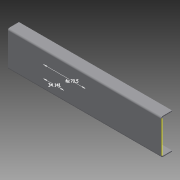
# Autodesk Inventor part: crane_lower
Saved by Autodesk Inventor 2014 SP2 (Build 180246200, 246)
## iProperties
Created: 2016-04-26
Part Number: crane_lower
Material: Generic
Document SubType Name: Sheet Metal
Designer: cruiser
Density: 1 g/cm^3
Flat Pattern Width: 9.17817 cm
Flat Pattern Length: 25.8 cm
Flat Pattern Area: 236.797 cm^2
Sheet Metal Rule: Default_mm
Sheet Metal Width: 91.782 mm
Sheet Metal Length: 258.000 mm
Sheet Metal Area: 23679.674 mm^2
Appearance: Default
Author: cruiser
Autodesk Inventor part; units mm, degrees
ref_plane "YZ Plane" through (0, 0, 0) normal (1, 0, 0) x (0, 1, 0)
ref_plane "XZ Plane" through (0, 0, 0) normal (0, 1, 0) x (-1, 0, 0)
ref_plane "XY Plane" through (0, 0, 0) normal (0, 0, 1) x (1, 0, 0)
sketch "Sketch1" plane through (0, 0, 0) normal (0, 1, 0) x (-1, 0, 0)
  line L0 (70.5, -70.5) -> (-70.5, -70.5)
  line L1 (-70.5, -70.5) -> (-70.5, 70.5)
  line L2 (-70.5, 70.5) -> (70.5, 70.5)
  line L3 (70.5, 70.5) -> (70.5, -70.5)
  line L4 (70.5, -70.5) -> (-70.5, 70.5) construction
  line L5 (-70.5, -70.5) -> (70.5, 70.5) construction
  line L6 (129, -30) -> (-129, -30)
  line L7 (-129, -30) -> (-129, 30)
  line L8 (-129, 30) -> (129, 30)
  line L9 (129, 30) -> (129, -30)
  line L10 (129, -30) -> (-129, 30) construction
  line L11 (-129, -30) -> (129, 30) construction
  point P0 (0, 0)
  dimension "d0" = 258
  dimension "d1" = 60
  dimension "d2" = 141
  dimension "d3" = 141
  measures "d0" distance of L6.start L6.end
  measures "d1" distance of L6.end L7.end
  measures "d2" distance of L0.start L0.end
  measures "d3" distance of L0.end L1.end
extrude "Plate1" add sketch "Sketch1" along normal blind 1.5875 contours L6 L1 L8 L3 | L3 L8 L9 L6 | L6 L7 L8 L1
sketch "Sketch4" plane through (129, 0, 28.4125) normal (0, 0, 1) x (1, 0, 0)
  line L0 (-258, 0) -> (0, 0)
  line L1 (0, 0) -> (0, 18.65)
  line L2 (0, 18.65) -> (-258, 18.65)
  line L3 (-258, 18.65) -> (-258, 0)
  constraints: 6 end point, 1 horizontal, 1 perpendicular, 1 vertical
edge flange "Flange3" height 18.65 angle 90 thickness 1.5875 bend radius 1.5875 thickness toward (0, 0, 1) relief straight relief width 1.5875 relief depth 0.7937 corner gap 1.5875 corner form 0 edges at (0, 1.5875, 30) (0, 1.5875, -30) wall of the first edge with corners at (-129, 0, 28.4125) (129, 0, 28.4125) (129, 18.65, 28.4125) (-129, 18.65, 28.4125)
bend "Bend3"
corner "Corner3"
sketch "Sketch5" plane through (0, 1.5875, 0) normal (0, 1, 0) x (1, 0, 0)
  line L0 (129, 26.825) -> (-129, 26.825) projected
  line L1 (-129, -26.825) -> (-129, 26.825) projected
  line L2 (-129, -26.825) -> (129, -26.825) projected
  line L3 (129, 26.825) -> (129, -26.825) projected
  line L4 (0, 26.825) -> (0, -26.825)
  line L5 (-70.5, 26.825) -> (-36.359, 26.825)
  line L6 (-36.359, 26.825) -> (-36.359, -26.825)
  line L7 (-36.359, -26.825) -> (-70.5, -26.825)
  line L8 (-70.5, -26.825) -> (-70.5, 26.825)
  line L9 (70.5, 26.825) -> (36.359, 26.825)
  line L10 (36.359, 26.825) -> (36.359, -26.825)
  line L11 (36.359, -26.825) -> (70.5, -26.825)
  line L12 (70.5, -26.825) -> (70.5, 26.825)
  point P0 (0, 0)
  dimension "d56" = 70.5
  dimension "d57" = 34.141
  constraints: 18 end point, 4 symmetric about line, 2 midpoint, 2 parallel, 2 point on line, 1 horizontal, 1 perpendicular
  measures "d56" distance between parallel lines of L4 L8
  measures "d57" distance between parallel lines of L6 L8
equation "\"d0\" = crane_x"
equation "\"d1\" = crane_y"
equation "\"d2\" = bed_x"
equation "\"d3\" = bed_y"
equation "\"d56\" = 0.5 * bed_x"
equation "\"Thickness\" = sm_thickness"
equation "\"d45\" = BendReliefWidth"
equation "\"d46\" = BendReliefDepth"
equation "\"d47\" = MinimumRemnant"
equation "\"d48\" = BendRadius"
equation "\"d49\" = crane_z - 4 * sm_thickness"
equation "\"d51\" = BendRadius"
equation "\"d52\" = CornerReliefSize"
equation "\"d53\" = GapSize"
equation "\"d54\" = JacobiRadiusSize"
equation "\"BendRadius\" = Thickness"
equation "\"BendReliefWidth\" = Thickness"
equation "\"BendReliefDepth\" = 0.5 * Thickness"
equation "\"CornerReliefSize\" = 4 * Thickness"
equation "\"MinimumRemnant\" = 2 * Thickness"
equation "\"TransitionRadius\" = BendRadius"
equation "\"JacobiRadiusSize\" = BendRadius"
equation "\"GapSize\" = Thickness"
equation "\"sm_thickness\" = 1.5875"
equation "\"thick_acrylic\" = 5.88"
equation "\"thin_acrylic\" = 3.15"
equation "\"clear_acrylic\" = 3.15"
equation "\"wood_thickness\" = 6.72"
equation "\"m3_diameter\" = 3.15"
equation "\"m4_diameter\" = 4.2"
equation "\"m5_diameter\" = 5.25"
equation "\"brass_insert_drill\" = 4"
equation "\"m5_brass_insert_drill\" = 6.7"
equation "\"m3_main_length\" = 14"
equation "\"m3_main_nut_width\" = 5.7"
equation "\"m3_main_nut_thickness\" = 2.5"
equation "\"m3_main_extra\" = 1"
equation "\"stepper_screw_space\" = 35"
equation "\"stepper_shaft_diameter\" = 5"
equation "\"stepper_body_diameter\" = 28"
equation "\"laser_body_diameter\" = 12"
equation "\"t_carrier\" = 5.88"
equation "\"t_wall\" = 5.88"
equation "\"t_window\" = 3.15"
equation "\"carrier_y\" = 181"
equation "\"carrier_z\" = 12"
equation "\"carrier_z2\" = 283.04"
equation "\"protection_slot\" = 36.2"
equation "\"protection_slot_offset\" = 45.25"
equation "\"protection_slot_length\" = 35"
equation "\"window_z\" = 185"
equation "\"window_y\" = 49.56"
equation "\"window_slot\" = 25"
equation "\"door_sensor\" = 35"
equation "\"reservoir_x\" = 151"
equation "\"reservoir_y\" = 151"
equation "\"reservoir_z\" = 25.4"
equation "\"reservoir_overlap\" = 5"
equation "\"linear_bearing_spacing\" = 207"
equation "\"linear_bearing_z\" = 304.8"
equation "\"threaded_rod_z\" = 203.2"
equation "\"motor_spacing\" = 287"
equation "\"t_tray\" = 3.15"
equation "\"tray_border\" = 15"
equation "\"tray_x\" = 181"
equation "\"tray_y\" = 181"
equation "\"bed_x\" = 141"
equation "\"bed_y\" = 141"
equation "\"brass_keep_out\" = 8"
equation "\"tape_keep_out\" = 2"
equation "\"tape_thickness\" = 2"
equation "\"t_crane\" = 6.72"
equation "\"crane_x\" = 258"
equation "\"crane_y\" = 60"
equation "\"crane_z\" = 25"
equation "\"end_stop_offset_x\" = 47"
equation "\"end_stop_spacing\" = 19"
equation "\"thumb_nut_offset_y\" = 11.72"
equation "\"thumb_nut_diameter\" = 7"
equation "\"z_min_from_center\" = 79"
equation "\"t_frame\" = 6.72"
equation "\"frame_top_z\" = 291"
equation "\"frame_bottom_z\" = 225"
equation "\"frame_total_z\" = 516"
equation "\"frame_y\" = 68.44"
equation "\"frame_border\" = 39.5"
equation "\"frame_foot_z\" = 49.5"
equation "\"frame_tilt\" = 1deg"
equation "\"printer_z\" = 289"
equation "\"lcd_x\" = 72"
equation "\"lcd_y\" = 25"
equation "\"subframe_y_offset\" = 27.5"
equation "\"laser_y_offset\" = 19.4"
equation "\"laser_diameter\" = 12"
equation "\"laser_z_offset\" = 55"
equation "\"laser_y\" = 35"
equation "\"laser_z\" = 18"
equation "\"laser_x\" = 24"
equation "\"t_galvo_frame\" = 6.72"
equation "\"galvo_frame_x\" = 66"
equation "\"galvo_frame_z\" = 65"
equation "\"galvo_frame_y_offset\" = 27.5"
equation "\"drawer_x\" = 181"
equation "\"drawer_y\" = 54.6925"
equation "\"drawer_z\" = 206.72"
equation "\"drawer_z_from_bottom\" = 25"
equation "\"d4\" = BendRadius"
equation "\"crane_z2\" = 12"
body "Solid1"
